OS from bioreactor base 3_v2 (Autodesk Fusion 360 design; units mm, degrees)
part number: Box Front
Autodesk Fusion 360 part; units mm, degrees
(part 1 of 5)
ref_plane "WorkPlane12" through (0, -1, 0) normal (0, 1, 0) x (0, 0, 1)
sketch "Box Big part" plane through (0, 0, 0) normal (0, 0, 1) x (1, 0, 0)
  line L0 (0, 0) -> (-240, 0)
  line L1 (-240, 0) -> (-240, 182)
  line L2 (-240, 182) -> (0, 182)
  line L3 (0, 182) -> (0, 0)
  line L4 (-240, 0) -> (-224.405, 0)
  line L5 (-224.405, 0) -> (-224.405, 3.175)
  line L6 (-224.405, 3.175) -> (-213.595, 3.175)
  line L7 (-213.595, 3.175) -> (-213.595, 0)
  circle A0 centre (-223.9829, 2.4679) radius 1
  circle A1 centre (-214.0171, 2.4679) radius 1
  line L8 (-240, 19.595) -> (-236.825, 19.595)
  line L9 (-236.825, 19.595) -> (-236.825, 30.405)
  line L10 (-236.825, 30.405) -> (-240, 30.405)
  circle A2 centre (-237.5321, 29.9829) radius 1
  circle A3 centre (-237.5321, 20.0171) radius 1
  line L11 (-288.405, 0) -> (-288.405, 3.175)
  line L12 (-302, 182) -> (-242, 182)
  line L13 (-242, 182) -> (-242, 0)
  line L14 (-288.405, 3.175) -> (-277.595, 3.175)
  circle A4 centre (-287.9829, 2.4679) radius 1
  line L15 (-277.595, 3.175) -> (-277.595, 0)
  circle A5 centre (-278.0171, 2.4679) radius 1
  line L16 (-302, 0) -> (-302, 182)
  line L17 (-242, 0) -> (-302, 0)
  line L18 (-245.175, 0) -> (-245.175, 19.405)
  line L19 (-245.175, 19.405) -> (-242, 19.405)
  line L20 (-242, 182) -> (-245.175, 182)
  line L21 (-245.175, 182) -> (-245.175, 162.595)
  line L22 (-245.175, 162.595) -> (-242, 162.595)
  line L23 (-242, 162.595) -> (-242, 182)
  line L24 (-242, 30.595) -> (-245.175, 30.595)
  line L25 (-245.175, 30.595) -> (-245.175, 41.405)
  line L26 (-245.175, 41.405) -> (-242, 41.405)
  line L27 (-242, 41.405) -> (-242, 30.595)
  circle A6 centre (-244.4679, 31.0171) radius 1
  circle A7 centre (-244.4679, 40.9829) radius 1
  circle A8 centre (-244.4679, 18.9829) radius 1
  line L28 (242, 48.595) -> (242, 62)
  line L29 (242, 62) -> (242, 2)
  line L30 (2, 2) -> (2, 62)
  line L31 (17.405, 5.175) -> (17.405, 2)
  line L32 (242, 37.405) -> (242, 26.595)
  line L33 (28.595, 2) -> (28.595, 5.175)
  line L34 (2, 2) -> (28.595, 2)
  line L35 (238.825, 15.405) -> (242, 15.405)
  line L36 (238.825, 48.595) -> (242, 48.595)
  line L37 (242, 2) -> (2, 2)
  line L38 (238.825, 26.595) -> (238.825, 37.405)
  line L39 (238.825, 62) -> (238.825, 48.595)
  circle A9 centre (29.0171, 4.4679) radius 1
  line L40 (2, 5.175) -> (17.405, 5.175)
  circle A10 centre (239.5321, 27.0171) radius 1
  line L41 (2, 62) -> (242, 62)
  line L42 (242, 62) -> (238.825, 62)
  line L43 (28.595, 5.175) -> (39.405, 5.175)
  circle A11 centre (16.9829, 4.4679) radius 1
  line L44 (238.825, 2) -> (238.825, 15.405)
  line L45 (238.825, 37.405) -> (242, 37.405)
  line L46 (39.405, 5.175) -> (39.405, 2)
  circle A12 centre (38.9829, 4.4679) radius 1
  line L47 (242, 26.595) -> (238.825, 26.595)
  circle A13 centre (239.5321, 36.9829) radius 1
  circle A14 centre (239.5321, 14.9829) radius 1
  line L48 (242, 5.175) -> (226.595, 5.175)
  line L49 (226.595, 5.175) -> (226.595, 2)
  circle A15 centre (-244.4679, 163.0171) radius 1
  circle A16 centre (227.0171, 4.4679) radius 1
  circle A17 centre (239.5321, 49.0171) radius 1
  line L50 (-272, 182) -> (-272, 0) construction
  circle A18 centre (-234, 346) radius 1.05
  circle A19 centre (-6, 346) radius 1.05
  line L51 (1.75, 0) -> (22.5, 0)
  dimension "d12" = 10.81
  dimension "d13" = 3.175
  dimension "d14" = 3.175
  dimension "d34" = 2
  dimension "d36" = 0.4221
  dimension "d37" = 0.7071
  dimension "d38" = 0.4221
  dimension "d48" = 2
  dimension "d49" = 0.4221
  dimension "d50" = 19.595
  dimension "d51" = 3.175
  dimension "d52" = 0.4221
  dimension "d54" = 0.7071
  dimension "d55" = 10.81
  dimension "d80" = 182
  dimension "d82" = 10.81
  dimension "d85" = 60
  dimension "d86" = 2
  dimension "d87" = 0.4221
  dimension "d88" = 0.7071
  dimension "d89" = 0.4221
  dimension "d98" = 2
  dimension "d99" = 19.405
  dimension "d100" = 3.175
  dimension "d104" = 3.175
  dimension "d105" = 10.81
  dimension "d113" = 2
  dimension "d114" = 0.7071
  dimension "d115" = 0.4221
  dimension "d116" = 2
  dimension "d117" = 0.4221
  dimension "d119" = 0.4221
  dimension "d122" = 13.595
  dimension "d140" = 60
  dimension "d141" = 10.81
  dimension "d142" = 3.175
  dimension "d143" = 3.175
  dimension "d144" = 240
  dimension "d145" = 2
  dimension "d146" = 0.4221
  dimension "d147" = 0.7071
  dimension "d148" = 0.4221
  dimension "d149" = 13.405
  dimension "d150" = 3.175
  dimension "d151" = 3.175
  dimension "d152" = 10.81
  dimension "d154" = 2
  dimension "d155" = 0.7071
  dimension "d156" = 0.4221
  dimension "d157" = 2
  dimension "d159" = 0.4221
  dimension "d160" = 3.175
  dimension "d163" = 2
  dimension "d164" = 0.4221
  dimension "d171" = 11.19
  dimension "d182" = 0.4221
  dimension "d183" = 3.175
  dimension "d184" = 2
  dimension "d185" = 2
  dimension "d186" = 0.4221
  dimension "d187" = 0.4221
  dimension "d189" = 15.595
  dimension "d191" = 15.405
  dimension "d192" = 11.19
  dimension "d193" = 15.405
  dimension "d354" = 11.19
  dimension "d416" = 0.4221
  dimension "d417" = 19.405
  dimension "d418" = 13.405
  dimension "d442" = 3.175
  dimension "d473" = 240
  dimension "d474" = 2
  dimension "d475" = 182
  dimension "d476" = 2
  constraint horizontal L0
  constraint vertical L1
  constraint horizontal L2
  constraint vertical L3
  constraint coincident L0.start L3.end
  constraint horizontal L4
  constraint perpendicular L4 L5
  constraint perpendicular L5 L6
  constraint perpendicular L6 L7
  constraint equal A0 A1
  constraint horizontal A0.centre A1.centre
  constraint coincident L1 L8.start
  constraint perpendicular L1 L8
  constraint perpendicular L8 L9
  constraint coincident L1 L10.end
  constraint perpendicular L1 L10
  constraint equal A2 A3
  constraint vertical A2.centre A3.centre
  constraint horizontal L17
  constraint vertical L16
  constraint horizontal L12
  constraint vertical L13
  constraint perpendicular L11 L14
  constraint perpendicular L14 L15
  constraint equal A4 A5
  constraint horizontal A4.centre A5.centre
  constraint coincident L17 L18.start
  constraint perpendicular L17 L18
  constraint coincident L13 L19.end
  constraint perpendicular L13 L19
  constraint horizontal L20
  constraint vertical L21
  constraint horizontal L22
  constraint vertical L23
  constraint horizontal L24
  constraint vertical L25
  constraint horizontal L26
  constraint vertical L27
  constraint coincident L13 L24.start
  constraint equal A6 A7
  constraint vertical A6.centre A7.centre
  constraint vertical A7.centre A8.centre
  constraint collinear L0 L17
  constraint horizontal L37
  constraint vertical L30
  constraint horizontal L41
  constraint vertical L29
  constraint horizontal L34
  constraint perpendicular L33 L34
  constraint perpendicular L33 L43
  constraint perpendicular L43 L46
  constraint equal A9 A12
  constraint horizontal A12.centre A9.centre
  constraint coincident L44.start L37
  constraint perpendicular L37 L44
  constraint coincident L35.end L29
  constraint perpendicular L29 L35
  constraint horizontal L42
  constraint vertical L39
  constraint horizontal L36
  constraint vertical L28
  constraint equal L35 L36
  constraint horizontal L47
  constraint vertical L38
  constraint horizontal L45
  constraint vertical L32
  constraint coincident L32.end L29
  constraint equal A10 A13
  constraint vertical A13.centre A10.centre
  constraint vertical A14.centre A13.centre
  constraint coincident L40.start L30
  constraint perpendicular L30 L40
  constraint coincident L31.end L34
  constraint perpendicular L31 L34
  constraint horizontal A9.centre A11.centre
  constraint coincident L29 L48.start
  constraint coincident L37 L49.end
  constraint perpendicular L37 L49
  constraint collinear L40 L48
  constraint vertical A7.centre A15.centre
  constraint equal A7 A15
  constraint horizontal A12.centre A16.centre
  constraint vertical A14.centre A17.centre
  constraint midpoint L12 L50.start
  constraint midpoint L17 L50.end
  constraint coincident L11.start L17
  measures "d12" distance of L5.end L6.end
  measures "d13" distance of L4.end L5.end
  measures "d14" distance of L6.end L7.end
  measures "d34" diameter of A0
  measures "d36" distance of L5 A0.centre
  measures "d37" distance of L6 A0.centre
  measures "d38" horizontal distance of L7.end A1.centre
  measures "d48" diameter of A2
  measures "d49" distance of L8 A3.centre
  measures "d50" distance of L4 L8
  measures "d51" distance of L9.end L10.end
  measures "d52" distance of L10 A2.centre
  measures "d54" distance of L9 A3.centre
  measures "d55" distance of L8 L10
  measures "d80" distance of L13.end L12.end
  measures "d82" distance of L11.end L14.end
  measures "d85" distance of L12.start L12.end
  measures "d86" diameter of A4
  measures "d87" distance of A4.centre L11
  measures "d88" distance of A4.centre L14
  measures "d89" horizontal distance of A5.centre L15.end
  measures "d98" distance of L0.end L13.end
  measures "d99" distance of L17 L19
  measures "d100" distance of L13 L18
  measures "d104" distance of L25.end L26.end
  measures "d105" distance of L24.end L25.end
  measures "d113" diameter of A6
  measures "d114" distance of L25 A6.centre
  measures "d115" distance of L24 A6.centre
  measures "d116" diameter of A8
  measures "d117" distance of L26 A7.centre
  measures "d119" distance of L19 A8.centre
  measures "d122" distance of L11 L16
  measures "d140" distance of L28.end L29.end
  measures "d141" distance of L43.end L33.end
  measures "d142" distance of L33.start L33.end
  measures "d143" distance of L43.end L46.end
  measures "d144" distance of L28.end L30.end
  measures "d145" diameter of A9
  measures "d146" distance of A9.centre L33
  measures "d147" distance of A9.centre L43
  measures "d148" horizontal distance of A12.centre L46.end
  measures "d149" distance of L35 L37
  measures "d150" distance of L29 L44
  measures "d151" distance of L38.end L32.start
  measures "d152" distance of L38.start L38.end
  measures "d154" diameter of A10
  measures "d155" distance of A10.centre L38
  measures "d156" distance of A10.centre L47
  measures "d157" diameter of A14
  measures "d159" distance of A14.centre L35
  measures "d160" distance of L34 L40
  measures "d163" diameter of A11
  measures "d164" distance of A11.centre L31
  measures "d171" distance of L35 L47
  measures "d182" vertical distance of L21.end A15.centre
  measures "d183" distance of L14 L17
  measures "d184" diameter of A17
  measures "d185" diameter of A16
  measures "d186" distance of L36 A17.centre
  measures "d187" distance of L49 A16.centre
  measures "d189" distance of L1 L5
  measures "d191" distance of L30 L31
  measures "d192" distance of L31 L33
  measures "d193" distance of L29 L49
  measures "d354" distance of L19 L24
  measures "d416" distance of A13.centre L45
  measures "d417" distance of L20.end L21.end
  measures "d418" distance of L36.start L39.start
  measures "d442" distance of L21.end L22.end
  measures "d473" distance of L1 L3
  measures "d474" distance of L3 L30
  measures "d475" distance of L0 L2
  measures "d476" distance of L37 L51
sketch "Box Medium part" plane through (0, 0, 0) normal (0, 0, 1) x (1, 0, 0)
  line L0 (28.095, 5.175) -> (38.905, 5.175)
  circle A0 centre (226.5171, 4.4679) radius 1
  line L1 (1.75, 0) -> (22.5, 0)
  line L2 (241.5, 37.405) -> (241.5, 26.595)
  line L3 (1.5, 2) -> (1.5, 62)
  line L4 (-0.5, 182) -> (-0.5, 0)
  line L5 (238.325, 15.405) -> (241.5, 15.405)
  line L6 (226.095, 5.175) -> (226.095, 2)
  line L7 (238.325, 2) -> (238.325, 15.405)
  line L8 (238.325, 62) -> (238.325, 48.595)
  circle A1 centre (16.4829, 4.4679) radius 1
  line L9 (241.5, 26.595) -> (238.325, 26.595)
  line L10 (1.5, 62) -> (241.5, 62)
  circle A2 centre (239.0321, 36.9829) radius 1
  line L11 (28.095, 2) -> (28.095, 5.175)
  circle A3 centre (239.0321, 14.9829) radius 1
  line L12 (-240.5, 182) -> (-0.5, 182)
  line L13 (-0.5, 0) -> (-240.5, 0)
  line L14 (-242.5, 182) -> (-245.675, 182)
  line L15 (-272.5, 182) -> (-272.5, 0) construction
  line L16 (-224.905, 0) -> (-224.905, 3.175)
  line L17 (-214.095, 3.175) -> (-214.095, 0)
  circle A4 centre (-214.5171, 2.4679) radius 1
  line L18 (-224.905, 3.175) -> (-214.095, 3.175)
  line L19 (-245.675, 182) -> (-245.675, 162.595)
  line L20 (-242.5, 30.595) -> (-245.675, 30.595)
  line L21 (-288.905, 3.175) -> (-278.095, 3.175)
  circle A5 centre (-238.0321, 29.9829) radius 1
  circle A6 centre (-244.9679, 40.9829) radius 1
  line L22 (-245.675, 0) -> (-245.675, 19.405)
  line L23 (-237.325, 19.595) -> (-237.325, 30.405)
  line L24 (-240.5, 19.595) -> (-237.325, 19.595)
  circle A7 centre (-238.0321, 20.0171) radius 1
  line L25 (-302.5, 0) -> (-302.5, 182)
  line L26 (-242.5, 0) -> (-302.5, 0)
  circle A8 centre (-278.5171, 2.4679) radius 1
  line L27 (241.5, 48.595) -> (241.5, 62)
  line L28 (238.325, 37.405) -> (241.5, 37.405)
  line L29 (1.5, 5.175) -> (16.905, 5.175)
  line L30 (38.905, 5.175) -> (38.905, 2)
  line L31 (-240.5, 0) -> (-240.5, 182)
  circle A9 centre (-244.9679, 163.0171) radius 1
  circle A10 centre (-244.9679, 18.9829) radius 1
  circle A11 centre (-224.4829, 2.4679) radius 1
  line L32 (-245.675, 162.595) -> (-242.5, 162.595)
  line L33 (-237.325, 30.405) -> (-240.5, 30.405)
  line L34 (-302.5, 182) -> (-242.5, 182)
  line L35 (-245.675, 30.595) -> (-245.675, 41.405)
  line L36 (-242.5, 41.405) -> (-242.5, 30.595)
  line L37 (241.5, 2) -> (1.5, 2)
  circle A12 centre (38.4829, 4.4679) radius 1
  line L38 (1.5, 2) -> (28.095, 2)
  line L39 (-242.5, 182) -> (-242.5, 0)
  line L40 (238.325, 48.595) -> (241.5, 48.595)
  circle A13 centre (-288.4829, 2.4679) radius 1
  circle A14 centre (-244.9679, 31.0171) radius 1
  line L41 (-245.675, 19.405) -> (-242.5, 19.405)
  circle A15 centre (28.5171, 4.4679) radius 1
  circle A16 centre (239.0321, 49.0171) radius 1
  line L42 (-242.5, 162.595) -> (-242.5, 182)
  line L43 (241.5, 62) -> (238.325, 62)
  line L44 (-288.905, 0) -> (-288.905, 3.175)
  line L45 (-240.5, 0) -> (-224.905, 0)
  line L46 (-278.095, 3.175) -> (-278.095, 0)
  line L47 (241.5, 62) -> (241.5, 2)
  line L48 (241.5, 5.175) -> (226.095, 5.175)
  line L49 (-245.675, 41.405) -> (-242.5, 41.405)
  circle A17 centre (239.0321, 27.0171) radius 1
  line L50 (238.325, 26.595) -> (238.325, 37.405)
  line L51 (16.905, 5.175) -> (16.905, 2)
  point P0 (-0.5, 0)
  dimension "d1796" = 10.81
  dimension "d1797" = 3.175
  dimension "d1798" = 3.175
  dimension "d1799" = 2
  dimension "d1800" = 0.4221
  dimension "d1801" = 0.7071
  dimension "d1802" = 0.4221
  dimension "d1803" = 2
  dimension "d1804" = 0.4221
  dimension "d1805" = 19.595
  dimension "d1806" = 3.175
  dimension "d1807" = 0.4221
  dimension "d1808" = 0.7071
  dimension "d1809" = 10.81
  dimension "d1810" = 182
  dimension "d1811" = 10.81
  dimension "d1812" = 60
  dimension "d1813" = 2
  dimension "d1814" = 0.4221
  dimension "d1815" = 0.7071
  dimension "d1816" = 0.4221
  dimension "d1817" = 2
  dimension "d1818" = 19.405
  dimension "d1819" = 3.175
  dimension "d1820" = 3.175
  dimension "d1821" = 10.81
  dimension "d1822" = 2
  dimension "d1823" = 0.7071
  dimension "d1824" = 0.4221
  dimension "d1825" = 2
  dimension "d1826" = 0.4221
  dimension "d1827" = 0.4221
  dimension "d1828" = 13.595
  dimension "d1829" = 60
  dimension "d1830" = 10.81
  dimension "d1831" = 3.175
  dimension "d1832" = 3.175
  dimension "d1833" = 240
  dimension "d1834" = 2
  dimension "d1835" = 0.4221
  dimension "d1836" = 0.7071
  dimension "d1837" = 0.4221
  dimension "d1838" = 13.405
  dimension "d1839" = 3.175
  dimension "d1840" = 3.175
  dimension "d1841" = 10.81
  dimension "d1842" = 2
  dimension "d1843" = 0.7071
  dimension "d1844" = 0.4221
  dimension "d1845" = 2
  dimension "d1846" = 0.4221
  dimension "d1847" = 3.175
  dimension "d1848" = 2
  dimension "d1849" = 0.4221
  dimension "d1850" = 11.19
  dimension "d1851" = 0.4221
  dimension "d1852" = 3.175
  dimension "d1853" = 2
  dimension "d1854" = 2
  dimension "d1855" = 0.4221
  dimension "d1856" = 0.4221
  dimension "d1857" = 15.595
  dimension "d1858" = 15.405
  dimension "d1859" = 11.19
  dimension "d1860" = 15.405
  dimension "d1861" = 11.19
  dimension "d1862" = 0.4221
  dimension "d1863" = 19.405
  dimension "d1864" = 13.405
  dimension "d1865" = 3.175
  dimension "d1866" = 240
  dimension "d1867" = 2
  dimension "d1868" = 182
  dimension "d1869" = 2
  constraint horizontal L13
  constraint vertical L31
  constraint horizontal L12
  constraint vertical L4
  constraint coincident P0 L4.end
  constraint horizontal L45
  constraint perpendicular L16 L45
  constraint perpendicular L16 L18
  constraint perpendicular L17 L18
  constraint equal A4 A11
  constraint horizontal A11.centre A4.centre
  constraint coincident L24.start L31
  constraint perpendicular L24 L31
  constraint perpendicular L23 L24
  constraint coincident L33.end L31
  constraint perpendicular L31 L33
  constraint equal A5 A7
  constraint vertical A5.centre A7.centre
  constraint horizontal L26
  constraint vertical L25
  constraint horizontal L34
  constraint vertical L39
  constraint perpendicular L21 L44
  constraint perpendicular L21 L46
  constraint equal A8 A13
  constraint horizontal A8.centre A13.centre
  constraint coincident L22.start L26
  constraint perpendicular L22 L26
  constraint coincident L41.end L39
  constraint perpendicular L39 L41
  constraint horizontal L14
  constraint vertical L19
  constraint horizontal L32
  constraint vertical L42
  constraint horizontal L20
  constraint vertical L35
  constraint horizontal L49
  constraint vertical L36
  constraint coincident L20.start L39
  constraint equal A6 A14
  constraint vertical A6.centre A14.centre
  constraint vertical A6.centre A10.centre
  constraint collinear L13 L26
  constraint horizontal L37
  constraint vertical L3
  constraint horizontal L10
  constraint vertical L47
  constraint horizontal L38
  constraint perpendicular L11 L38
  constraint perpendicular L0 L11
  constraint perpendicular L0 L30
  constraint equal A12 A15
  constraint horizontal A12.centre A15.centre
  constraint coincident L7.start L37
  constraint perpendicular L7 L37
  constraint coincident L5.end L47
  constraint perpendicular L5 L47
  constraint horizontal L43
  constraint vertical L8
  constraint horizontal L40
  constraint vertical L27
  constraint equal L5 L40
  constraint horizontal L9
  constraint vertical L50
  constraint horizontal L28
  constraint vertical L2
  constraint coincident L2.end L47
  constraint equal A2 A17
  constraint vertical A2.centre A17.centre
  constraint vertical A2.centre A3.centre
  constraint coincident L29.start L3
  constraint perpendicular L3 L29
  constraint coincident L51.end L38
  constraint perpendicular L38 L51
  constraint horizontal A1.centre A15.centre
  constraint coincident L48.start L47
  constraint coincident L6.end L37
  constraint perpendicular L6 L37
  constraint collinear L29 L48
  constraint vertical A6.centre A9.centre
  constraint equal A6 A9
  constraint horizontal A12.centre A0.centre
  constraint vertical A3.centre A16.centre
  constraint midpoint L15.start L34
  constraint midpoint L15.end L26
  constraint coincident L44.start L26
  measures "d1796" distance of L16.end L17.start
  measures "d1797" distance of L16.start L16.end
  measures "d1798" distance of L17.end L17.start
  measures "d1799" diameter of A11
  measures "d1800" distance of A11.centre L16
  measures "d1801" distance of A11.centre L18
  measures "d1802" horizontal distance of L17.end A4.centre
  measures "d1803" diameter of A5
  measures "d1804" distance of A7.centre L24
  measures "d1805" distance of L24 L45
  measures "d1806" distance of L33.end L23.end
  measures "d1807" distance of A5.centre L33
  measures "d1808" distance of A7.centre L23
  measures "d1809" distance of L24 L33
  measures "d1810" distance of L26.start L14.start
  measures "d1811" distance of L21.end L21.start
  measures "d1812" distance of L25.end L14.start
  measures "d1813" diameter of A13
  measures "d1814" distance of A13.centre L44
  measures "d1815" distance of A13.centre L21
  measures "d1816" horizontal distance of A8.centre L46.end
  measures "d1817" distance of L13.end L26.start
  measures "d1818" distance of L26 L41
  measures "d1819" distance of L22 L39
  measures "d1820" distance of L36.start L35.end
  measures "d1821" distance of L20.end L35.end
  measures "d1822" diameter of A14
  measures "d1823" distance of A14.centre L35
  measures "d1824" distance of A14.centre L20
  measures "d1825" diameter of A10
  measures "d1826" distance of A6.centre L49
  measures "d1827" distance of A10.centre L41
  measures "d1828" distance of L25 L44
  measures "d1829" distance of L10.end L37.start
  measures "d1830" distance of L0.end L0.start
  measures "d1831" distance of L11.start L0.start
  measures "d1832" distance of L30.end L0.end
  measures "d1833" distance of L3.end L10.end
  measures "d1834" diameter of A15
  measures "d1835" distance of A15.centre L11
  measures "d1836" distance of A15.centre L0
  measures "d1837" horizontal distance of L30.end A12.centre
  measures "d1838" distance of L5 L37
  measures "d1839" distance of L7 L47
  measures "d1840" distance of L28.start L2.start
  measures "d1841" distance of L9.end L28.start
  measures "d1842" diameter of A17
  measures "d1843" distance of A17.centre L50
  measures "d1844" distance of A17.centre L9
  measures "d1845" diameter of A3
  measures "d1846" distance of A3.centre L5
  measures "d1847" distance of L29 L38
  measures "d1848" diameter of A1
  measures "d1849" distance of A1.centre L51
  measures "d1850" distance of L5 L9
  measures "d1851" vertical distance of L19.end A9.centre
  measures "d1852" distance of L21 L26
  measures "d1853" diameter of A16
  measures "d1854" diameter of A0
  measures "d1855" distance of A16.centre L40
  measures "d1856" distance of A0.centre L6
  measures "d1857" distance of L16 L31
  measures "d1858" distance of L3 L51
  measures "d1859" distance of L11 L51
  measures "d1860" distance of L6 L47
  measures "d1861" distance of L20 L41
  measures "d1862" distance of A2.centre L28
  measures "d1863" distance of L19.end L14.end
  measures "d1864" distance of L8.start L8.end
  measures "d1865" distance of L19.end L32.end
  measures "d1866" distance of L4 L31
  measures "d1867" distance of L3 L4
  measures "d1868" distance of L12 L13
  measures "d1869" distance of L1 L37
sketch "Box Small Part" plane through (0, 0, 0) normal (0, 0, 1) x (1, 0, 0)
  line L0 (-288.405, 0) -> (-288.405, 1.5613)
  line L1 (-245.175, 0) -> (-245.175, 18.2758)
  line L2 (-243.5613, 41.405) -> (-242, 41.405)
  line L3 (-287.2758, 3.175) -> (-278.7242, 3.175)
  line L4 (-277.595, 1.5613) -> (-277.595, 0)
  line L5 (-243.5613, 19.405) -> (-242, 19.405)
  line L6 (-242, 30.595) -> (-242, 19.405)
  arc A0 (-243.5613, 19.405) -> (-245.175, 18.2758) centre (-244.4679, 18.9829) ccw
  arc A1 (-245.175, 31.7242) -> (-243.5613, 30.595) centre (-244.4679, 31.0171) ccw
  line L7 (-242, 30.595) -> (-243.5613, 30.595)
  line L8 (-245.175, 31.7242) -> (-245.175, 40.2758)
  arc A2 (-243.5613, 41.405) -> (-245.175, 40.2758) centre (-244.4679, 40.9829) ccw
  line L9 (-266.405, 0) -> (-277.595, 0)
  line L10 (-288.405, 0) -> (-298.825, 0)
  arc A3 (-287.2758, 3.175) -> (-288.405, 1.5613) centre (-287.9829, 2.4679) ccw
  arc A4 (-277.595, 1.5613) -> (-278.7242, 3.175) centre (-278.0171, 2.4679) ccw
  line L11 (-242, 52.595) -> (-242, 41.405)
  line L12 (-394.5485, 91) -> (-201, 91) construction
  arc A5 (-245.175, 163.7242) -> (-243.5613, 162.595) centre (-244.4679, 163.0171) ccw
  line L13 (-245.175, 182) -> (-245.175, 163.7242)
  line L14 (-243.5613, 162.595) -> (-242, 162.595)
  line L15 (1.75, 0) -> (22.5, 0)
  line L16 (-272, -12.9167) -> (-272, 179) construction
  line L17 (0, 1.75) -> (0, 22.5)
  arc A6 (-245.175, 163.7242) -> (-243.5613, 162.595) centre (-244.4679, 163.0171) ccw
  line L18 (-243.5613, 162.595) -> (-242, 162.595)
  line L19 (-245.175, 182) -> (-245.175, 163.7242)
  line L20 (-242, 151.405) -> (-242, 162.595)
  line L21 (-298.825, 31.7242) -> (-298.825, 40.2758)
  line L22 (-298.825, 0) -> (-298.825, 18.2758)
  line L23 (-302, 30.595) -> (-302, 19.405)
  arc A7 (-298.825, 18.2758) -> (-300.4387, 19.405) centre (-299.5321, 18.9829) ccw
  line L24 (-302, 52.595) -> (-302, 41.405)
  line L25 (-300.4387, 19.405) -> (-302, 19.405)
  line L26 (-300.4387, 41.405) -> (-302, 41.405)
  line L27 (-302, 30.595) -> (-300.4387, 30.595)
  arc A8 (-298.825, 40.2758) -> (-300.4387, 41.405) centre (-299.5321, 40.9829) ccw
  arc A9 (-300.4387, 30.595) -> (-298.825, 31.7242) centre (-299.5321, 31.0171) ccw
  line L28 (-277.595, 180.4387) -> (-277.595, 182)
  line L29 (-287.2758, 178.825) -> (-278.7242, 178.825)
  line L30 (-266.405, 182) -> (-277.595, 182)
  arc A10 (-288.405, 180.4387) -> (-287.2758, 178.825) centre (-287.9829, 179.5321) ccw
  line L31 (-288.405, 182) -> (-288.405, 180.4387)
  arc A11 (-278.7242, 178.825) -> (-277.595, 180.4387) centre (-278.0171, 179.5321) ccw
  line L32 (-288.405, 182) -> (-298.825, 182)
  line L33 (-302, 151.405) -> (-302, 162.595)
  arc A12 (-300.4387, 162.595) -> (-298.825, 163.7242) centre (-299.5321, 163.0171) ccw
  line L34 (-300.4387, 162.595) -> (-302, 162.595)
  line L35 (-298.825, 182) -> (-298.825, 163.7242)
  arc A13 (-300.4387, 162.595) -> (-298.825, 163.7242) centre (-299.5321, 163.0171) ccw
  line L36 (-300.4387, 162.595) -> (-302, 162.595)
  line L37 (-298.825, 182) -> (-298.825, 163.7242)
  line L38 (-242, 74.595) -> (-242, 63.405)
  line L39 (-245.175, 53.7242) -> (-245.175, 62.2758)
  line L40 (-242, 52.595) -> (-243.5613, 52.595)
  line L41 (-243.5613, 63.405) -> (-242, 63.405)
  arc A14 (-245.175, 53.7242) -> (-243.5613, 52.595) centre (-244.4679, 53.0171) ccw
  arc A15 (-243.5613, 63.405) -> (-245.175, 62.2758) centre (-244.4679, 62.9829) ccw
  line L42 (-242, 96.595) -> (-242, 85.405)
  line L43 (-245.175, 75.7242) -> (-245.175, 84.2758)
  line L44 (-242, 74.595) -> (-243.5613, 74.595)
  line L45 (-243.5613, 85.405) -> (-242, 85.405)
  arc A16 (-245.175, 75.7242) -> (-243.5613, 74.595) centre (-244.4679, 75.0171) ccw
  arc A17 (-243.5613, 85.405) -> (-245.175, 84.2758) centre (-244.4679, 84.9829) ccw
  line L46 (-242, 118.595) -> (-242, 107.405)
  line L47 (-245.175, 97.7242) -> (-245.175, 106.2758)
  line L48 (-242, 96.595) -> (-243.5613, 96.595)
  line L49 (-243.5613, 107.405) -> (-242, 107.405)
  arc A18 (-245.175, 97.7242) -> (-243.5613, 96.595) centre (-244.4679, 97.0171) ccw
  arc A19 (-243.5613, 107.405) -> (-245.175, 106.2758) centre (-244.4679, 106.9829) ccw
  line L50 (-242, 140.595) -> (-242, 129.405)
  line L51 (-245.175, 119.7242) -> (-245.175, 128.2758)
  line L52 (-242, 118.595) -> (-243.5613, 118.595)
  line L53 (-243.5613, 129.405) -> (-242, 129.405)
  arc A20 (-245.175, 119.7242) -> (-243.5613, 118.595) centre (-244.4679, 119.0171) ccw
  arc A21 (-243.5613, 129.405) -> (-245.175, 128.2758) centre (-244.4679, 128.9829) ccw
  line L54 (-242, 162.595) -> (-242, 151.405)
  line L55 (-245.175, 141.7242) -> (-245.175, 150.2758)
  line L56 (-242, 140.595) -> (-243.5613, 140.595)
  line L57 (-243.5613, 151.405) -> (-242, 151.405)
  arc A22 (-245.175, 141.7242) -> (-243.5613, 140.595) centre (-244.4679, 141.0171) ccw
  arc A23 (-243.5613, 151.405) -> (-245.175, 150.2758) centre (-244.4679, 150.9829) ccw
  line L58 (-300.4387, 63.405) -> (-302, 63.405)
  arc A24 (-300.4387, 52.595) -> (-298.825, 53.7242) centre (-299.5321, 53.0171) ccw
  arc A25 (-298.825, 62.2758) -> (-300.4387, 63.405) centre (-299.5321, 62.9829) ccw
  line L59 (-298.825, 53.7242) -> (-298.825, 62.2758)
  line L60 (-302, 52.595) -> (-300.4387, 52.595)
  line L61 (-302, 74.595) -> (-302, 63.405)
  line L62 (-300.4387, 85.405) -> (-302, 85.405)
  arc A26 (-300.4387, 74.595) -> (-298.825, 75.7242) centre (-299.5321, 75.0171) ccw
  arc A27 (-298.825, 84.2758) -> (-300.4387, 85.405) centre (-299.5321, 84.9829) ccw
  line L63 (-298.825, 75.7242) -> (-298.825, 84.2758)
  line L64 (-302, 74.595) -> (-300.4387, 74.595)
  line L65 (-302, 96.595) -> (-302, 85.405)
  line L66 (-300.4387, 107.405) -> (-302, 107.405)
  arc A28 (-300.4387, 96.595) -> (-298.825, 97.7242) centre (-299.5321, 97.0171) ccw
  arc A29 (-298.825, 106.2758) -> (-300.4387, 107.405) centre (-299.5321, 106.9829) ccw
  line L67 (-298.825, 97.7242) -> (-298.825, 106.2758)
  line L68 (-302, 96.595) -> (-300.4387, 96.595)
  line L69 (-302, 118.595) -> (-302, 107.405)
  line L70 (-300.4387, 129.405) -> (-302, 129.405)
  arc A30 (-300.4387, 118.595) -> (-298.825, 119.7242) centre (-299.5321, 119.0171) ccw
  arc A31 (-298.825, 128.2758) -> (-300.4387, 129.405) centre (-299.5321, 128.9829) ccw
  line L71 (-298.825, 119.7242) -> (-298.825, 128.2758)
  line L72 (-302, 118.595) -> (-300.4387, 118.595)
  line L73 (-302, 140.595) -> (-302, 129.405)
  line L74 (-300.4387, 151.405) -> (-302, 151.405)
  arc A32 (-300.4387, 140.595) -> (-298.825, 141.7242) centre (-299.5321, 141.0171) ccw
  arc A33 (-298.825, 150.2758) -> (-300.4387, 151.405) centre (-299.5321, 150.9829) ccw
  line L75 (-298.825, 141.7242) -> (-298.825, 150.2758)
  line L76 (-302, 140.595) -> (-300.4387, 140.595)
  line L77 (-302, 162.595) -> (-302, 151.405)
  arc A34 (-265.2758, 3.175) -> (-266.405, 1.5613) centre (-265.9829, 2.4679) ccw
  line L78 (-265.2758, 3.175) -> (-256.7242, 3.175)
  line L79 (-244.405, 0) -> (-255.595, 0)
  line L80 (-266.405, 0) -> (-266.405, 1.5613)
  line L81 (-255.595, 1.5613) -> (-255.595, 0)
  arc A35 (-255.595, 1.5613) -> (-256.7242, 3.175) centre (-256.0171, 2.4679) ccw
  line L82 (-244.405, 182) -> (-255.595, 182)
  line L83 (-255.595, 180.4387) -> (-255.595, 182)
  line L84 (-266.405, 182) -> (-266.405, 180.4387)
  arc A36 (-266.405, 180.4387) -> (-265.2758, 178.825) centre (-265.9829, 179.5321) ccw
  line L85 (-265.2758, 178.825) -> (-256.7242, 178.825)
  arc A37 (-256.7242, 178.825) -> (-255.595, 180.4387) centre (-256.0171, 179.5321) ccw
  line L86 (-245.175, 0) -> (-245.945, 0)
  line L87 (-245.175, 182) -> (-244.405, 182)
  dimension "d1887" = 2
  dimension "d1888" = 0.4221
  dimension "d1889" = 0.7071
  dimension "d1890" = 0.4221
  dimension "d1896" = 2
  dimension "d1899" = 2
  dimension "d1926" = 3.175
  dimension "d1948" = 0.7071
  dimension "d1949" = 0.4221
  dimension "d1951" = 0.4221
  dimension "d1953" = 10.81
  dimension "d1956" = 11.19
  dimension "d1958" = 0.4221
  dimension "d1959" = 0.7071
  dimension "d1960" = 0.7071
  dimension "d1961" = 10.81
  dimension "d1962" = 11.19
  dimension "d1963" = 242
  dimension "d1965" = 3.175
  dimension "d1974" = 91
  dimension "d1975" = 19.405
  dimension "d1976" = 11.19
  dimension "d1979" = 91
  dimension "d1984" = 272
  dimension "d1989" = 13.595
  dimension "d1992" = 22
  dimension "d1993" = 22
  dimension "d1996" = 0
  dimension "d1997" = 22
  dimension "d2000" = 0
  dimension "d2001" = 22
  dimension "d2004" = 22
  dimension "d2005" = 0
  dimension "d2008" = 22
  dimension "d2009" = 0
  dimension "d2010" = -0.77
  constraint horizontal L9
  constraint perpendicular L0 L3
  constraint perpendicular L3 L4
  constraint equal A3 A4
  constraint horizontal A4.centre A3.centre
  constraint perpendicular L1 L9
  constraint equal A1 A2
  constraint coincident L0.start L9
  constraint perpendicular L6 L7
  constraint collinear L9 L10
  constraint perpendicular L5 L11
  constraint vertical L8
  constraint collinear L1 L8
  constraint collinear L6 L11
  constraint horizontal L12
  constraint symmetric L5.end L12 L14.end
  constraint symmetric L1.start L12 L13.start
  constraint symmetric L1.end L12 A5.start
  constraint symmetric L5.start L12 A5.end
  constraint symmetric A0 L12 A5
  constraint collinear L10 L15
  constraint vertical L16
  constraint symmetric L6.start L12 L20.start
  constraint symmetric A0 L12 A6
  constraint symmetric L5.end L16 L23.end
  constraint symmetric L2.end L16 L24.end
  constraint symmetric L6.start L16 L23.start
  constraint symmetric L1.start L16 L10.end
  constraint symmetric L1.end L16 L22.end
  constraint symmetric L5.start L16 A7.end
  constraint symmetric A0 L16 A7
  constraint symmetric A1.end L16 L27.end
  constraint symmetric A1.start L16 L21.start
  constraint symmetric A1 L16 A9
  constraint symmetric L8.end L16 L21.end
  constraint symmetric L2.start L16 L26.start
  constraint symmetric A2 L16 A8
  constraint symmetric L11.start L16 L24.start
  constraint symmetric L0.start L12 L31.start
  constraint symmetric L4.end L12 L28.end
  constraint symmetric L0.end L12 A10.start
  constraint symmetric L3.start L12 L29.start
  constraint symmetric A3 L12 A10
  constraint symmetric L3.end L12 L29.end
  constraint symmetric L4.start L12 L28.start
  constraint symmetric A4 L12 A11
  constraint symmetric L12 L9.start L30.start
  constraint symmetric L12 L10.end L32.end
  constraint symmetric L13.start L16 L32.end
  constraint symmetric A5.start L16 A12.end
  constraint symmetric L14.end L16 L33.end
  constraint symmetric A5.end L16 A12.start
  constraint symmetric A5 L16 A12
  constraint symmetric L16 L13.start L32.end
  constraint symmetric L16 A5.start A12.end
  constraint symmetric L16 L14.end L33.end
  constraint symmetric L16 A5.end A12.start
  constraint symmetric L16 A6 A13
  constraint symmetric L16 L20.start L33.start
  constraint perpendicular L1 L86
  constraint perpendicular L13 L87
  constraint equal L86 L87
  measures "d1887" diameter of A3
  measures "d1888" distance of A3.centre L0
  measures "d1889" distance of A3.centre L3
  measures "d1890" horizontal distance of A4.centre L4.end
  measures "d1896" diameter of A1
  measures "d1899" diameter of A0
  measures "d1926" distance of L3 L9
  measures "d1948" distance of A0.centre L1
  measures "d1949" distance of A0.centre L5
  measures "d1951" distance of A1.centre L7
  measures "d1953" distance of L2 L7
  measures "d1956" distance of L5 A1.end
  measures "d1958" distance of A2.centre L2
  measures "d1959" distance of A1.centre L8
  measures "d1960" distance of A2.centre L8
  measures "d1961" distance of L0 L4
  measures "d1962" distance of L2 L11.start
  measures "d1963" distance of origin L6
  measures "d1965" distance of L6 L8
  measures "d1974" vertical distance of origin L12.end
  measures "d1975" distance of L1.start L5
  measures "d1976" distance of L4.end L9.start
  measures "d1979" vertical distance of L1.start L12.end
  measures "d1984" distance of L16 L17
  measures "d1989" distance of L0 L23
  measures "d2010" distance of L1.start L86.end
sketch "MyStock" plane through (0, 0, 0) normal (0, 0, 1) x (1, 0, 0)
  line L0 (-332.6683, 184.6624) -> (156, 184.6624)
  line L1 (156, 184.6624) -> (156, -91)
  line L2 (156, -91) -> (-332.6683, -91)
  line L3 (-332.6683, -91) -> (-332.6683, 184.6624)
  constraint horizontal L0
  constraint vertical L1
  constraint horizontal L2
  constraint vertical L3
extrude "Extrude19" add sketch "MyStock" along normal blind 3.175
extrude "Top" [suppressed]
pattern_linear "Top length repeat holes" [suppressed]
pattern_linear "Top depth repeat holes" [suppressed]
ref_plane "WorkPlane5" through (-107.5475, 91, 1.5875) normal (0, -1, 0) x (1, 0, 0)
mirror "Mirror Bottom on X" [suppressed]
combine "Combine5" [suppressed]
ref_plane "WorkPlane6" through (-120, 91, 1.5875) normal (1, 0, 0) x (0, 1, 0)
mirror "Mirror Bottom on Y" [suppressed]
combine "FInish Top" [suppressed]
mirror "Create Bottom" [suppressed]
extrude "Right" [suppressed]
pattern_linear "Right height repeat holes" [suppressed]
pattern_linear "Right depth repeat holes" [suppressed]
ref_plane "WorkPlane7" through (-261.135, 91, 1.5875) normal (0, -1, 0) x (1, 0, 0)
mirror "Mirror Right on X" [suppressed]
combine "Combine7" [suppressed]
ref_plane "WorkPlane8" through (-272, 91, 1.5875) normal (-1, 0, 0) x (0, 1, 0)
mirror "Mirror10" [suppressed]
combine "Finish Right" [suppressed]
mirror "Create Left" [suppressed]
extrude "Front" [suppressed]
pattern_linear "Front length repeat holes" [suppressed]
pattern_linear "Front height repeat holes" [suppressed]
ref_plane "WorkPlane9" through (132, 32, 1.5875) normal (0, -1, 0) x (1, 0, 0)
mirror "Mirror Front on X" [suppressed]
combine "Combine9" [suppressed]
ref_plane "WorkPlane11" through (122, 32, 1.5875) normal (-1, 0, 0) x (0, -1, 0)
mirror "Mirror12" [suppressed]
combine "Finish Front" [suppressed]
mirror "Create Back" [suppressed]
sketch "Box Stock sketch" plane through (0, 0, 0) normal (0, 0, 1) x (1, 0, 0)
  line L0 (0, -184) -> (-304.8, -184)
  line L1 (-304.8, -184) -> (-304.8, 425.6)
  line L2 (-304.8, 425.6) -> (0, 425.6)
  line L3 (0, 425.6) -> (0, -184)
  line L4 (1.75, 0) -> (22.5, 0)
  line L5 (0, 1.75) -> (0, 22.5)
  dimension "d206" = 304.8
  dimension "d207" = 609.6
  dimension "d1621" = 184
  constraint horizontal L0
  constraint vertical L1
  constraint horizontal L2
  constraint vertical L3
  constraint collinear L3 L5
  measures "d206" distance of L0.start L0.end
  measures "d207" distance of L0.end L1.end
  measures "d1621" distance of L0 L4
copy_body "Body->Comp1" [suppressed] in component "Top"
copy_body "Body->Comp9" [suppressed] in component "Bottom"
copy_body "Body->Comp8" [suppressed] in component "Front"
copy_body "Body->Comp10" [suppressed] in component "Back"
copy_body "Body->Comp7" [suppressed] in component "Right"
copy_body "Body->Comp11" [suppressed] in component "Left"